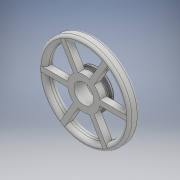
# Autodesk Inventor part: 뒷바퀴2
Saved by Autodesk Inventor 2018 (Build 220112000, 112)
## iProperties
Created: 2019-11-13
Part Number: 뒷바퀴2
Material: 일반
Document SubType Name: Modeling
Designer: LeeYounSeo
Density: 1 g/cm^3
Appearance: 기본값
Author: LeeYounSeo
Autodesk Inventor part; units mm, degrees
ref_plane "YZ Plane" through (0, 0, 0) normal (1, 0, 0) x (0, 1, 0)
ref_plane "XZ Plane" through (0, 0, 0) normal (0, 1, 0) x (-1, 0, 0)
ref_plane "XY Plane" through (0, 0, 0) normal (0, 0, 1) x (1, 0, 0)
sketch "스케치1" plane through (0, 0, 0) normal (0, 1, 0) x (-1, 0, 0)
  circle A0 centre (0, 0) radius 7.5
  circle A1 centre (0, 0) radius 10
  dimension "d0" = 15
  dimension "d1" = 20
  constraints: 2 centre point, 2 coincident
  measures "d0" diameter of A0
  measures "d1" diameter of A1
extrude "돌출1" add sketch "스케치1" along normal blind 4.5
sketch "스케치2" plane through (0, 4.5, 0) normal (0, 1, 0) x (1, 0, 0)
  circle A0 centre (0, 0) radius 13.5
  circle A1 centre (0, 0) radius 10 projected
  circle A2 centre (0, 0) radius 7.5 projected
  circle A3 centre (0, 0) radius 10 projected
  dimension "d4" = 27
  constraints: 1 centre point, 1 coincident
  measures "d4" diameter of A0
extrude "돌출2" add sketch "스케치2" against normal blind 1 contours A0 | A1
sketch "스케치3" plane through (0, 0, 0) normal (0, -1, 0) x (1, 0, 0)
  circle A0 centre (0, 0) radius 14
  circle A1 centre (0, 0) radius 7.5 projected
  circle A2 centre (0, 0) radius 10 projected
  dimension "d7" = 28
  constraints: 1 centre point, 1 coincident
  measures "d7" diameter of A0
extrude "돌출3" add sketch "스케치3" against normal blind 1 contours A0 | A2
sketch "스케치4" plane through (0, 0, 0) normal (0, -1, 0) x (1, 0, 0)
  circle A0 centre (0, 0) radius 12.5
  circle A1 centre (0, 0) radius 14 projected
  circle A2 centre (0, 0) radius 7.5 projected
  dimension "d10" = 25
  constraints: 1 centre point, 1 coincident
  measures "d10" diameter of A0
extrude "돌출4" add sketch "스케치4" along normal blind 5 contours A0
sketch "스케치5" plane through (0, -5, 0) normal (0, -1, 0) x (1, 0, 0)
  circle A0 centre (0, 0) radius 35
  circle A1 centre (0, 0) radius 30
  dimension "d13" = 70
  dimension "d14" = 60
  constraints: 2 centre point, 2 coincident
  measures "d13" diameter of A0
  measures "d14" diameter of A1
extrude "돌출5" add sketch "스케치5" against normal blind 5
sketch "스케치6" plane through (0, 0, 0) normal (0, 1, 0) x (1, 0, 0)
  circle A0 centre (0, 0) radius 30 projected
  circle A1 centre (0, 0) radius 35 projected
extrude "돌출6" add sketch "스케치6" along normal blind 3
sketch "스케치7" plane through (0, -5, 0) normal (0, -1, 0) x (1, 0, 0)
  line L0 (32.5, 2) -> (-32.5, 2)
  line L1 (-32.5, 2) -> (-32.5, -2)
  line L2 (-32.5, -2) -> (32.5, -2)
  line L3 (32.5, -2) -> (32.5, 2)
  point P0 (0, 0)
  dimension "d19" = 4
  dimension "d20" = 65
  dimension "d21" = 2
  dimension "d22" = 32.5
  constraints: 8 end point, 2 parallel, 1 horizontal, 1 perpendicular
  measures "d19" distance of L0.end L1.end
  measures "d20" distance of L1.end L2.end
  measures "d21" distance from line of point (0, 0) L2
  measures "d22" distance from line of point (0, 0) L3
extrude "돌출7" add sketch "스케치7" against normal blind 5
pattern_circular "원형 패턴1" count 6 over 360 about axis through (0, 0, 0) along (0, -1, 0) of "돌출7"
sketch "스케치8" plane through (0, -5, 0) normal (0, -1, 0) x (1, 0, 0)
  circle A0 centre (0, 0) radius 7.5
  dimension "d28" = 15
  constraints: 1 centre point, 1 coincident
  measures "d28" diameter of A0
extrude "돌출8" cut sketch "스케치8" against normal blind 10
fillet "모깎기1" radius 2 2 edges at (-35, 3, 0) (-35, -5, 0)
fillet "모깎기2" radius 0.8 2 edges at (-13.5, 3.5, 0) (-14, 1, 0)
fillet "모깎기3" radius 3 7 edges at (-30, 3, 0) (-25.9808, -5, -15) (-25.9808, -5, 15) (0, -5, 30) (0, -5, -30) (25.9808, -5, 15) (25.9808, -5, -15) curvature continuous yes
